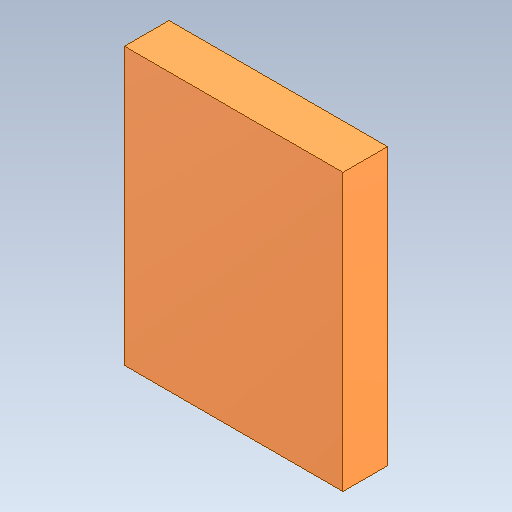
# Autodesk Inventor part: LM358MX
Saved by Autodesk Inventor 2021 (Build 250183000, 183)
## iProperties
Created: 2020-11-18
Part Number: LM358MX
Material: Generic
Document SubType Name: Modeling
Designer: Admin
Density: 1 g/cm^3
Appearance: SO08, LM358MX
Author: Admin
Autodesk Inventor part; units mm, degrees
ref_plane "YZ Plane" through (0, 0, 0) normal (1, 0, 0) x (0, 1, 0)
ref_plane "XZ Plane" through (0, 0, 0) normal (0, 1, 0) x (-1, 0, 0)
ref_plane "XY Plane" through (0, 0, 0) normal (0, 0, 1) x (1, 0, 0)
sketch "SO08, LM358MX_22" plane through (0, 0, 0) normal (0, 0, 1) x (1, 0, 0)
  line L0 (-2.4, 3.1) -> (2.5016, 3.1)
  line L1 (2.5016, 3.1) -> (2.5016, -3.1)
  line L2 (2.5016, -3.1) -> (-2.4, -3.1)
  line L3 (-2.4, -3.1) -> (-2.4, 3.1)
  constraints: 8 end point
extrude "Extrusion1" add sketch "SO08, LM358MX_22" along normal blind 1
body "Solid1"
